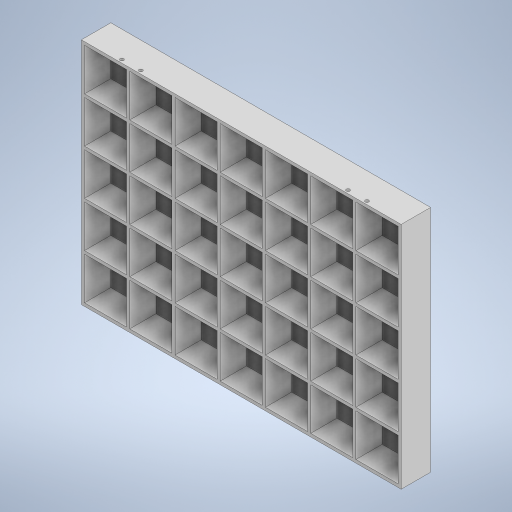
# Autodesk Inventor part: RatPelletBox_v04
Saved by Autodesk Inventor 2024 (Build 280153000, 153)
## iProperties
Created: 2025-06-19
Part Number: RatPelletBox_v04
Material: Generic
Document SubType Name: Modeling
Designer: Akramilab
Density: 1 g/cm^3
Appearance: Default
Author: Akramilab
Autodesk Inventor part; units mm, degrees
ref_plane "YZ Plane" through (0, 0, 0) normal (1, 0, 0) x (0, 1, 0)
ref_plane "XZ Plane" through (0, 0, 0) normal (0, 1, 0) x (-1, 0, 0)
ref_plane "XY Plane" through (0, 0, 0) normal (0, 0, 1) x (1, 0, 0)
sketch "Sketch1" plane through (0, 0, 0) normal (0, 0, 1) x (1, 0, 0)
  line L0 (-152, -109) -> (152, -109)
  line L1 (152, -109) -> (152, 109)
  line L2 (152, 109) -> (-152, 109)
  line L3 (-152, 109) -> (-152, -109)
  line L4 (-152, -109) -> (152, 109) construction
  line L5 (152, -109) -> (-152, 109) construction
  point P0 (0, 0)
  dimension "d0" = 304
  dimension "d1" = 218
  constraints: 12 end point, 2 midpoint, 2 parallel, 1 horizontal, 1 perpendicular
  measures "d0" distance of L1.end L2.end
  measures "d1" distance of L0.end L1.end
extrude "Extrusion1" add sketch "Sketch1" along normal blind 28
sketch "Sketch2" plane through (0, 0, 28) normal (0, 0, 1) x (1, 0, 0)
  line L0 (-149, 106) -> (-109, 106)
  line L1 (-109, 106) -> (-109, 66)
  line L2 (-109, 66) -> (-149, 66)
  line L3 (-149, 66) -> (-149, 106)
  line L4 (-149, 106) -> (-109, 66) construction
  line L5 (-109, 106) -> (-149, 66) construction
  line L6 (152, 109) -> (-152, 109) projected
  line L7 (-152, 109) -> (-152, -109) projected
  line L8 (-106, 106) -> (-66, 106)
  line L9 (-66, 106) -> (-66, 66)
  line L10 (-66, 66) -> (-106, 66)
  line L11 (-106, 66) -> (-106, 106)
  line L12 (-106, 106) -> (-66, 66) construction
  line L13 (-66, 106) -> (-106, 66) construction
  line L14 (-63, 106) -> (-23, 106)
  line L15 (-23, 106) -> (-23, 66)
  line L16 (-23, 66) -> (-63, 66)
  line L17 (-63, 66) -> (-63, 106)
  line L18 (-63, 106) -> (-23, 66) construction
  line L19 (-23, 106) -> (-63, 66) construction
  line L20 (-20, 106) -> (20, 106)
  line L21 (20, 106) -> (20, 66)
  line L22 (20, 66) -> (-20, 66)
  line L23 (-20, 66) -> (-20, 106)
  line L24 (-20, 106) -> (20, 66) construction
  line L25 (20, 106) -> (-20, 66) construction
  line L26 (23, 106) -> (63, 106)
  line L27 (63, 106) -> (63, 66)
  line L28 (63, 66) -> (23, 66)
  line L29 (23, 66) -> (23, 106)
  line L30 (23, 106) -> (63, 66) construction
  line L31 (63, 106) -> (23, 66) construction
  line L32 (-149, 63) -> (-109, 63)
  line L33 (-109, 63) -> (-109, 23)
  line L34 (-109, 23) -> (-149, 23)
  line L35 (-149, 23) -> (-149, 63)
  line L36 (-149, 63) -> (-109, 23) construction
  line L37 (-109, 63) -> (-149, 23) construction
  line L38 (-106, 63) -> (-66, 63)
  line L39 (-66, 63) -> (-66, 23)
  line L40 (-66, 23) -> (-106, 23)
  line L41 (-106, 23) -> (-106, 63)
  line L42 (-106, 63) -> (-66, 23) construction
  line L43 (-66, 63) -> (-106, 23) construction
  line L44 (-63, 63) -> (-23, 63)
  line L45 (-23, 63) -> (-23, 23)
  line L46 (-23, 23) -> (-63, 23)
  line L47 (-63, 23) -> (-63, 63)
  line L48 (-63, 63) -> (-23, 23) construction
  line L49 (-23, 63) -> (-63, 23) construction
  line L50 (-20, 63) -> (20, 63)
  line L51 (20, 63) -> (20, 23)
  line L52 (20, 23) -> (-20, 23)
  line L53 (-20, 23) -> (-20, 63)
  line L54 (-20, 63) -> (20, 23) construction
  line L55 (20, 63) -> (-20, 23) construction
  line L56 (23, 63) -> (63, 63)
  line L57 (63, 63) -> (63, 23)
  line L58 (63, 23) -> (23, 23)
  line L59 (23, 23) -> (23, 63)
  line L60 (23, 63) -> (63, 23) construction
  line L61 (63, 63) -> (23, 23) construction
  line L62 (-149, 20) -> (-109, 20)
  line L63 (-109, 20) -> (-109, -20)
  line L64 (-109, -20) -> (-149, -20)
  line L65 (-149, -20) -> (-149, 20)
  line L66 (-149, 20) -> (-109, -20) construction
  line L67 (-109, 20) -> (-149, -20) construction
  line L68 (-106, 20) -> (-66, 20)
  line L69 (-66, 20) -> (-66, -20)
  line L70 (-66, -20) -> (-106, -20)
  line L71 (-106, -20) -> (-106, 20)
  line L72 (-106, 20) -> (-66, -20) construction
  line L73 (-66, 20) -> (-106, -20) construction
  line L74 (-63, 20) -> (-23, 20)
  line L75 (-23, 20) -> (-23, -20)
  line L76 (-23, -20) -> (-63, -20)
  line L77 (-63, -20) -> (-63, 20)
  line L78 (-63, 20) -> (-23, -20) construction
  line L79 (-23, 20) -> (-63, -20) construction
  line L80 (-20, 20) -> (20, 20)
  line L81 (20, 20) -> (20, -20)
  line L82 (20, -20) -> (-20, -20)
  line L83 (-20, -20) -> (-20, 20)
  line L84 (-20, 20) -> (20, -20) construction
  line L85 (20, 20) -> (-20, -20) construction
  line L86 (23, 20) -> (63, 20)
  line L87 (63, 20) -> (63, -20)
  line L88 (63, -20) -> (23, -20)
  line L89 (23, -20) -> (23, 20)
  line L90 (23, 20) -> (63, -20) construction
  line L91 (63, 20) -> (23, -20) construction
  line L92 (-149, -23) -> (-109, -23)
  line L93 (-109, -23) -> (-109, -63)
  line L94 (-109, -63) -> (-149, -63)
  line L95 (-149, -63) -> (-149, -23)
  line L96 (-149, -23) -> (-109, -63) construction
  line L97 (-109, -23) -> (-149, -63) construction
  line L98 (-106, -23) -> (-66, -23)
  line L99 (-66, -23) -> (-66, -63)
  line L100 (-66, -63) -> (-106, -63)
  line L101 (-106, -63) -> (-106, -23)
  line L102 (-106, -23) -> (-66, -63) construction
  line L103 (-66, -23) -> (-106, -63) construction
  line L104 (-63, -23) -> (-23, -23)
  line L105 (-23, -23) -> (-23, -63)
  line L106 (-23, -63) -> (-63, -63)
  line L107 (-63, -63) -> (-63, -23)
  line L108 (-63, -23) -> (-23, -63) construction
  line L109 (-23, -23) -> (-63, -63) construction
  line L110 (-20, -23) -> (20, -23)
  line L111 (20, -23) -> (20, -63)
  line L112 (20, -63) -> (-20, -63)
  line L113 (-20, -63) -> (-20, -23)
  line L114 (-20, -23) -> (20, -63) construction
  line L115 (20, -23) -> (-20, -63) construction
  line L116 (23, -23) -> (63, -23)
  line L117 (63, -23) -> (63, -63)
  line L118 (63, -63) -> (23, -63)
  line L119 (23, -63) -> (23, -23)
  line L120 (23, -23) -> (63, -63) construction
  line L121 (63, -23) -> (23, -63) construction
  line L122 (66, 106) -> (106, 106)
  line L123 (106, 106) -> (106, 66)
  line L124 (106, 66) -> (66, 66)
  line L125 (66, 66) -> (66, 106)
  line L126 (66, 106) -> (106, 66) construction
  line L127 (106, 106) -> (66, 66) construction
  line L128 (66, 63) -> (106, 63)
  line L129 (106, 63) -> (106, 23)
  line L130 (106, 23) -> (66, 23)
  line L131 (66, 23) -> (66, 63)
  line L132 (66, 63) -> (106, 23) construction
  line L133 (106, 63) -> (66, 23) construction
  line L134 (66, 20) -> (106, 20)
  line L135 (106, 20) -> (106, -20)
  line L136 (106, -20) -> (66, -20)
  line L137 (66, -20) -> (66, 20)
  line L138 (66, 20) -> (106, -20) construction
  line L139 (106, 20) -> (66, -20) construction
  line L140 (66, -23) -> (106, -23)
  line L141 (106, -23) -> (106, -63)
  line L142 (106, -63) -> (66, -63)
  line L143 (66, -63) -> (66, -23)
  line L144 (66, -23) -> (106, -63) construction
  line L145 (106, -23) -> (66, -63) construction
  line L146 (109, 106) -> (149, 106)
  line L147 (149, 106) -> (149, 66)
  line L148 (149, 66) -> (109, 66)
  line L149 (109, 66) -> (109, 106)
  line L150 (109, 106) -> (149, 66) construction
  line L151 (149, 106) -> (109, 66) construction
  line L152 (109, 63) -> (149, 63)
  line L153 (149, 63) -> (149, 23)
  line L154 (149, 23) -> (109, 23)
  line L155 (109, 23) -> (109, 63)
  line L156 (109, 63) -> (149, 23) construction
  line L157 (149, 63) -> (109, 23) construction
  line L158 (109, 20) -> (149, 20)
  line L159 (149, 20) -> (149, -20)
  line L160 (149, -20) -> (109, -20)
  line L161 (109, -20) -> (109, 20)
  line L162 (109, 20) -> (149, -20) construction
  line L163 (149, 20) -> (109, -20) construction
  line L164 (109, -23) -> (149, -23)
  line L165 (149, -23) -> (149, -63)
  line L166 (149, -63) -> (109, -63)
  line L167 (109, -63) -> (109, -23)
  line L168 (109, -23) -> (149, -63) construction
  line L169 (149, -23) -> (109, -63) construction
  line L170 (-149, -66) -> (-109, -66)
  line L171 (-109, -66) -> (-109, -106)
  line L172 (-109, -106) -> (-149, -106)
  line L173 (-149, -106) -> (-149, -66)
  line L174 (-149, -66) -> (-109, -106) construction
  line L175 (-109, -66) -> (-149, -106) construction
  line L176 (-106, -66) -> (-66, -66)
  line L177 (-66, -66) -> (-66, -106)
  line L178 (-66, -106) -> (-106, -106)
  line L179 (-106, -106) -> (-106, -66)
  line L180 (-106, -66) -> (-66, -106) construction
  line L181 (-66, -66) -> (-106, -106) construction
  line L182 (-63, -66) -> (-23, -66)
  line L183 (-23, -66) -> (-23, -106)
  line L184 (-23, -106) -> (-63, -106)
  line L185 (-63, -106) -> (-63, -66)
  line L186 (-63, -66) -> (-23, -106) construction
  line L187 (-23, -66) -> (-63, -106) construction
  line L188 (-20, -66) -> (20, -66)
  line L189 (20, -66) -> (20, -106)
  line L190 (20, -106) -> (-20, -106)
  line L191 (-20, -106) -> (-20, -66)
  line L192 (-20, -66) -> (20, -106) construction
  line L193 (20, -66) -> (-20, -106) construction
  line L194 (23, -66) -> (63, -66)
  line L195 (63, -66) -> (63, -106)
  line L196 (63, -106) -> (23, -106)
  line L197 (23, -106) -> (23, -66)
  line L198 (23, -66) -> (63, -106) construction
  line L199 (63, -66) -> (23, -106) construction
  line L200 (66, -66) -> (106, -66)
  line L201 (106, -66) -> (106, -106)
  line L202 (106, -106) -> (66, -106)
  line L203 (66, -106) -> (66, -66)
  line L204 (66, -66) -> (106, -106) construction
  line L205 (106, -66) -> (66, -106) construction
  line L206 (109, -66) -> (149, -66)
  line L207 (149, -66) -> (149, -106)
  line L208 (149, -106) -> (109, -106)
  line L209 (109, -106) -> (109, -66)
  line L210 (109, -66) -> (149, -106) construction
  line L211 (149, -66) -> (109, -106) construction
  point P0 (0, 0)
  point P1 (-129, 86)
  point P2 (-86, 86)
  point P3 (-43, 86)
  point P4 (0, 86)
  point P5 (43, 86)
  point P6 (-129, 43)
  point P7 (-86, 43)
  point P8 (-43, 43)
  point P9 (0, 43)
  point P10 (43, 43)
  point P11 (-129, 0)
  point P12 (-86, 0)
  point P13 (-43, 0)
  point P14 (0, 0)
  point P15 (43, 0)
  point P16 (-129, -43)
  point P17 (-86, -43)
  point P18 (-43, -43)
  point P19 (0, -43)
  point P20 (43, -43)
  point P21 (86, 86)
  point P22 (86, 43)
  point P23 (86, 0)
  point P24 (86, -43)
  point P25 (129, 86)
  point P26 (129, 43)
  point P27 (129, 0)
  point P28 (129, -43)
  point P29 (-129, -86)
  point P30 (-86, -86)
  point P31 (-43, -86)
  point P32 (0, -86)
  point P33 (43, -86)
  point P34 (86, -86)
  point P35 (129, -86)
  dimension "d4" = 40
  dimension "d5" = 3
  dimension "d6" = 3
  dimension "d7" = 40
  dimension "d10" = 43
  dimension "d13" = 43
  constraints: 420 end point, 2 collinear, 2 horizontal, 2 midpoint, 2 parallel, 1 perpendicular, 1 vertical, 372 other
  measures "d4" distance of L0.start L0.end
  measures "d5" distance between parallel lines of L6 L0
  measures "d6" distance between parallel lines of L7 L3
  measures "d7" distance of L0.end L1.end
  measures "d10" distance of L0.start L8.start
  measures "d13" distance of L0.start L32.start
extrude "Extrusion2" cut sketch "Sketch2" against normal blind 25
sketch "Sketch3" plane through (-152, 109, 0) normal (0, 1, 0) x (1, 0, 0)
  line L0 (46, -28) -> (46, -3) construction
  line L1 (43, -28) -> (43, -3) construction
  line L2 (43, -28) -> (43, -3) projected
  line L3 (43, -25) -> (46, -25) construction
  line L4 (46, -28) -> (46, -3) projected
  line L5 (304, -28) -> (0, -28) projected
  circle A0 centre (53.5, -25) radius 1.65
  circle A1 centre (35.5, -25) radius 1.65
  line L6 (172, -28) -> (172, -3) construction
  line L7 (175, -28) -> (175, -3) construction
  circle A2 centre (268.5, -25) radius 1.65
  circle A3 centre (250.5, -25) radius 1.65
  line L8 (304, 0) -> (304, -28) projected
  point P0 (152, 0)
  point P1 (44.5, -25)
  dimension "d20" = 3
  dimension "d21" = 3.3
  dimension "d22" = 9
  dimension "d23" = 3.3
  dimension "d24" = 9
  dimension "d25" = 3.3
  dimension "d31" = 3.3
  dimension "d35" = 18
  dimension "d36" = 35.5
  constraints: 4 centre point, 4 point on line, 2 end point, 1 midpoint, 1 perpendicular
  measures "d20" distance from line of L5 point (44.5, -25)
  measures "d21" diameter of A0
  measures "d22" distance of A0.centre point (44.5, -25)
  measures "d23" diameter of A1
  measures "d24" distance of A1.centre point (44.5, -25)
  measures "d25" diameter of A2
  measures "d31" diameter of A3
  measures "d35" distance of A2.centre A3.centre
  measures "d36" distance from line of A2.centre L8
extrude "Extrusion3" cut sketch "Sketch3" against normal blind 10
equation "\"d0\" = box_length"
equation "\"d1\" = box_width"
equation "\"d2\" = hole_height + wall"
equation "\"d4\" = hole"
equation "\"d5\" = wall"
equation "\"d6\" = wall"
equation "\"d7\" = hole"
equation "\"d10\" = hole + wall"
equation "\"d13\" = hole + wall"
equation "\"d16\" = hole_height"
equation "\"d23\" = d21"
equation "\"d24\" = d22"
equation "\"d25\" = d21"
equation "\"d31\" = d25"
equation "\"hole\" = 40"
equation "\"wall\" = 3"
equation "\"hole_height\" = 25"
equation "\"box_length\" = 304"
equation "\"box_width\" = 218"
body "Solid1"
